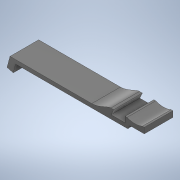
# Autodesk Inventor part: bat_lock02
Saved by Autodesk Inventor 2020 (Build 240168000, 168)
## iProperties
Created: 2023-12-19
Part Number: bat_lock02
Material: Типовые
Document SubType Name: Modeling
Designer: denis
Density: 1 g/cm^3
Appearance: По умолчанию
Author: denis
Autodesk Inventor part; units mm, degrees
ref_plane "YZ Plane" through (0, 0, 0) normal (1, 0, 0) x (0, 1, 0)
ref_plane "XZ Plane" through (0, 0, 0) normal (0, 1, 0) x (-1, 0, 0)
ref_plane "XY Plane" through (0, 0, 0) normal (0, 0, 1) x (1, 0, 0)
sketch "Эскиз1" plane through (0, 0, 0) normal (0, 0, 1) x (1, 0, 0)
  line L0 (0, 0) -> (1, 0)
  line L1 (10, 0) -> (10, -3)
  line L2 (10, -3) -> (3, -3)
  line L3 (0, -3) -> (0, 0)
  line L4 (0, -3) -> (-7.3989, -3)
  line L5 (-7.3989, -3) -> (-7.3989, -5) construction
  line L6 (-7.3989, -5) -> (0, -5)
  line L7 (0, -5) -> (0, -3) construction
  line L8 (0, -3) -> (2, -3) construction
  line L9 (2, -4) -> (2, -4)
  line L10 (1, -5) -> (0, -5)
  line L11 (0, -5) -> (0, -3) construction
  line L12 (-7.3989, -3) -> (-6, 0)
  line L13 (-7.3989, -3) -> (-13.5, -3) construction
  line L14 (-57.3989, -3) -> (-57.3989, -5) construction
  line L15 (-57.3989, -5) -> (-7.3989, -5)
  line L16 (-7.3989, -5) -> (-7.3989, -3) construction
  arc A0 (1, -5) -> (2, -4) centre (1, -4) ccw
  arc A1 (3, -3) -> (2, -4) centre (3, -4) ccw
  line L17 (-13.5, -3) -> (-17.5, -3) construction
  line L18 (0, 0) -> (1, 0)
  line L19 (10, 0) -> (9, 0)
  arc A2 (1, 0) -> (9, 0) centre (5, 9.1652) ccw
  line L20 (-57.3989, -3) -> (-60.318, -3)
  line L21 (-60.318, -3) -> (-62.6373, -11.6555)
  line L22 (-62.6373, -12.7273) -> (-58.6373, -12.7273) construction
  line L23 (-58.6373, -12.7273) -> (-58.6373, -9.6215) construction
  line L24 (-58.6373, -12.7273) -> (4.3374, -29.6013)
  line L25 (4.3374, -29.6013) -> (5.1139, -26.7036)
  line L26 (5.1139, -26.7036) -> (-58.6373, -9.6215)
  line L27 (-58.6373, -9.6215) -> (-58.6373, -12.7273) construction
  line L28 (-57.3989, -5) -> (-57.3989, -3) construction
  line L29 (-58.6373, -9.6215) -> (-57.3989, -5)
  line L30 (-13.5, -3) -> (-17.5, -3) construction
  line L31 (-17.5, -3) -> (-57.3989, -3)
  line L32 (1, 0) -> (9, 0) construction
  line L33 (9, 0) -> (10, 0)
  line L34 (-58.6373, -12.7273) -> (-62.6373, -11.6555)
  line L35 (-62.6373, -11.6555) -> (-62.6373, -12.7273) construction
  line L36 (-6, 0) -> (-7.5, 0) construction
  line L37 (-7.5, 0) -> (-7.5, -3) construction
  line L38 (-7.5, 0) -> (-9.5, 0) construction
  line L39 (-7.5, 0) -> (-9.5, 0) construction
  line L40 (-9.5, 0) -> (-13.5, -3) construction
  line L41 (-13.5, -3) -> (-17.5, -3) construction
  spline S0 degree 3 poles (-7.5, 0) (-9.5, 0) (-13.5, -3) (-17.5, -3) knots 1 1 1 1 2 2 2 2
  line L42 (-7.5, 0) -> (-6, 0)
  point P0 (2, -5)
  point P1 (0, -5)
  dimension "d0" = 10
  dimension "d1" = 3
  dimension "d3" = 2
  dimension "d4" = 2
  dimension "d5" = 2
  dimension "d6" = 50
  dimension "d9" = 1
  dimension "d10" = 1
  dimension "d11" = 4
  dimension "d13" = 2
  dimension "d14" = 1
  dimension "d15" = 1
  dimension "d16" = 10
  dimension "d17" = 4
  dimension "d18" = 10
  dimension "d20" = 3
  dimension "d21" = 65.1962
  dimension "d25" = 4.7845
  dimension "d26" = 66
  dimension "d27" = 90
  dimension "d28" = 105
  dimension "d29" = 65
  dimension "d30" = 6
  dimension "d31" = 3
  dimension "d32" = 1.5
  dimension "d33" = 6
  dimension "d34" = 2
  constraints: 80 end point, 17 parallel, 11 horizontal, 11 perpendicular, 7 point on line, 6 point on circle, 4 collinear, 4 tangent, 3 centre point, 2 coincident, 3 other
  measures "d0" distance of L1.end L3.start
  measures "d1" distance of L1.start L1.end
  measures "d3" distance of L5.end L4.end
  measures "d4" distance of point (2, -5) L10.end
  measures "d5" distance of L8.end point (2, -5)
  measures "d6" distance of L15.end L14.end
  measures "d9" radius of A0
  measures "d10" radius of A1
  measures "d11" distance of L13.end L17.end
  measures "d13" distance between parallel lines of L13 L15
  measures "d14" distance of L0.start L0.end
  measures "d15" distance of L1.start L19.end
  measures "d16" radius of A2
  measures "d17" distance of L22.end L22.start
  measures "d18" distance of L22.start L20.end
  measures "d20" distance of L25.end L24.end
  measures "d21" distance of L22.end L24.end
  measures "d25" distance of L23.end L14.end
  measures "d26" distance of L25.end L23.end
  measures "d27" angle of L29 L26
  measures "d28" angle of L20 L21
  measures "d29" angle of L12 L4
  measures "d30" distance from line of L12.end L3
  measures "d31" distance from line of L4 L12.end
  measures "d32" distance of L12.end L36.end
  measures "d33" distance from line of L13.end L37
  measures "d34" distance of L36.end L38.end
extrude "Выдавливание1" add sketch "Эскиз1" along normal blind 15
sketch "Эскиз3" plane through (0, 0, 15) normal (0, 0, 1) x (1, 0, 0)
  line L0 (-57.3989, -5) -> (1, -5) construction
  arc A0 (1, -5) -> (2, -4) centre (1, -4) ccw construction
  arc A1 (3, -3) -> (2, -4) centre (3, -4) ccw construction
  line L1 (3, -3) -> (10, -3) construction
  line L2 (10, -3) -> (10, 0) construction
  line L3 (10, 0) -> (9, 0) construction
  arc A2 (1, 0) -> (9, 0) centre (5, 9.1652) ccw construction
  line L4 (1, 0) -> (0, 0) construction
  line L5 (0, 0) -> (0, -3) construction
  line L6 (0, -3) -> (-7.3989, -3) construction
  line L7 (-7.3989, -3) -> (-6, 0) construction
  line L8 (-6, 0) -> (-7.5, 0) construction
  line L9 (-17.5, -3) -> (-60.318, -3) construction
  line L10 (-60.318, -3) -> (-62.6373, -11.6555) construction
  line L11 (-62.6373, -11.6555) -> (4.3374, -29.6013) construction
  line L12 (4.3374, -29.6013) -> (5.1139, -26.7036) construction
  line L13 (5.1139, -26.7036) -> (-58.6373, -9.6215) construction
  line L14 (-58.6373, -9.6215) -> (-57.3989, -5) construction
  line L15 (5.1139, -26.7036) -> (-58.6373, -9.6215) construction
  line L16 (-58.6373, -9.6215) -> (-61.8608, -8.7578)
  line L17 (-58.6373, -9.6215) -> (9.5, -23.7826)
  line L18 (9.5, -23.7826) -> (5.9363, -35.0214)
  line L19 (5.9363, -35.0214) -> (-67.9626, -14.6873)
  line L20 (-67.9626, -14.6873) -> (-64.2581, -8.4533)
  line L21 (-64.2581, -8.4533) -> (-61.8608, -8.7578)
  constraints: 12 end point, 2 point on line, 1 perpendicular, 1 other
extrude "Выдавливание2" cut sketch "Эскиз3" against normal blind 25
